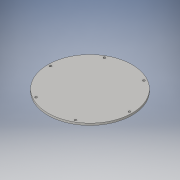
# Autodesk Inventor part: Back Lens
Saved by Autodesk Inventor 2016 (Build 200138000, 138)
## iProperties
Created: 2017-10-13
Part Number: Back Lens
Material: Generic
Document SubType Name: Modeling
Designer: Student
Density: 1 g/cm^3
Appearance: Default
Author: Student
Autodesk Inventor part; units mm, degrees
ref_plane "YZ Plane" through (0, 0, 0) normal (1, 0, 0) x (0, 1, 0)
ref_plane "XZ Plane" through (0, 0, 0) normal (0, 1, 0) x (-1, 0, 0)
ref_plane "XY Plane" through (0, 0, 0) normal (0, 0, 1) x (1, 0, 0)
sketch "Sketch1" plane through (0, 0, 0) normal (0, 1, 0) x (-1, 0, 0)
  circle A0 centre (0, 0) radius 58.801
  circle A1 centre (55.245, 0) radius 1.5
  circle A2 centre (27.6225, 47.8436) radius 1.5
  circle A3 centre (-27.6225, 47.8436) radius 1.5
  circle A4 centre (-55.245, 0) radius 1.5
  circle A5 centre (-27.6225, -47.8436) radius 1.5
  circle A6 centre (27.6225, -47.8436) radius 1.5
  dimension "d0" = 117.602
  dimension "d1" = 3
  dimension "d2" = 55.245
  dimension "d5" = 360
  constraints: 7 centre point, 1 coincident, 13 other
  measures "d0" diameter of A0
  measures "d1" diameter of A1
  measures "d2" distance of A1.centre point (0, 0)
extrude "Extrusion1" add sketch "Sketch1" along normal blind 2.7432
body "Solid1"
